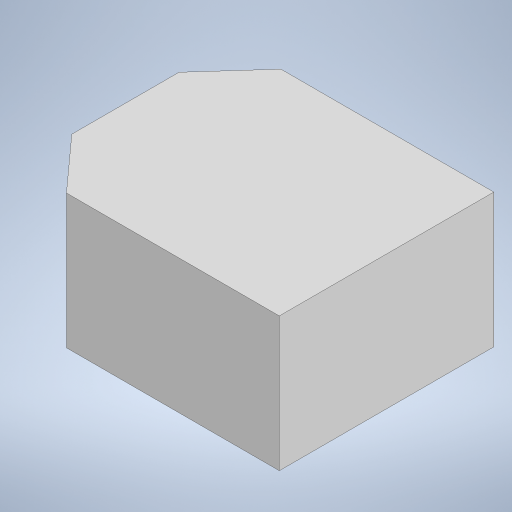
# Autodesk Inventor part: Część1
Saved by Autodesk Inventor 2023 (Build 270158000, 158)
## iProperties
Created: 2024-04-17
Part Number: Część1
Material: Ogólny
Document SubType Name: Modeling
Designer: domin
Density: 1 g/cm^3
Appearance: Domyślna
Author: domin
Autodesk Inventor part; units mm, degrees
ref_plane "YZ Plane" through (0, 0, 0) normal (1, 0, 0) x (0, 1, 0)
ref_plane "XZ Plane" through (0, 0, 0) normal (0, 1, 0) x (-1, 0, 0)
ref_plane "XY Plane" through (0, 0, 0) normal (0, 0, 1) x (1, 0, 0)
sketch "Szkic1" plane through (0, 0, 0) normal (0, 1, 0) x (-1, 0, 0)
  line L0 (0, 0) -> (0, -40)
  line L1 (0, 0) -> (39.7, 0)
  line L2 (0, -40) -> (39.7, -40)
  line L3 (48.7, -10) -> (48.7, -30)
  line L4 (48.7, -10) -> (39.7, 0)
  line L5 (48.7, -30) -> (39.7, -40)
  point P0 (48.7, -20)
  point P1 (0, -20)
  dimension "d0" = 40
  dimension "d1" = 39.7
  dimension "d3" = 20
  dimension "d6" = 138.013
  dimension "d7" = 138.013
  dimension "d8" = 48.7
  constraints: 12 end point, 2 horizontal, 2 midpoint, 1 parallel, 1 vertical
  measures "d0" distance of L0.start L0.end
  measures "d1" distance of L0.start L1.end
  measures "d3" distance of L3.start L3.end
  measures "d6" angle of L4 L3
  measures "d7" angle of L3 L5
  measures "d8" distance between parallel lines of L3 L0
extrude "Wyciągnięcie proste1" add sketch "Szkic1" along normal blind 25
